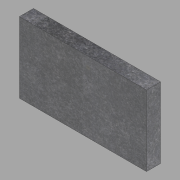
# Autodesk Inventor part: 4-1x-54x30x6 sn step
Saved by Autodesk Inventor 2022.1 (Build 261234020, 234B)
## iProperties
Created: 2021-11-03
Part Number: 4-1x-54x30x6 sn step
Material: Granite, Cut, Polished
Document SubType Name: Modeling
Designer: awelt
Density: 2.7 g/cm^3
Appearance: Kasota SN sapphire
Mass: 430062 g
Surface Area: 27406.4 cm^2
Volume: 159282 cm^3
Author: awelt
Autodesk Inventor part; units mm, degrees
ref_plane "YZ Plane" through (0, 0, 0) normal (1, 0, 0) x (0, 1, 0)
ref_plane "XZ Plane" through (0, 0, 0) normal (0, 1, 0) x (-1, 0, 0)
ref_plane "XY Plane" through (0, 0, 0) normal (0, 0, 1) x (1, 0, 0)
sketch "Sketch1" plane through (0, 0, 0) normal (0, 0, 1) x (1, 0, 0)
  line L0 (-685.8, 381) -> (685.8, 381)
  line L1 (685.8, 381) -> (685.8, -381)
  line L2 (685.8, -381) -> (-685.8, -381)
  line L3 (-685.8, -381) -> (-685.8, 381)
  line L4 (-685.8, 381) -> (685.8, -381) construction
  line L5 (685.8, 381) -> (-685.8, -381) construction
  point P0 (0, 0)
  dimension "d0" = 1371.6
  dimension "d1" = 762
  constraints: 12 end point, 2 midpoint, 2 parallel, 1 horizontal, 1 perpendicular
  measures "d0" distance of L1.end L2.end
  measures "d1" distance of L0.end L1.end
extrude "Extrusion1" add sketch "Sketch1" along normal blind 152.4
body "Solid1"
